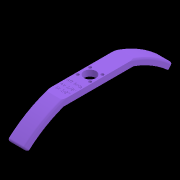
# Autodesk Inventor part: aft_holes
Saved by Autodesk Inventor 2020.2 (Build 242310000, 310)
## iProperties
Created: 2020-04-29
Part Number: aft_holes
Material: PC/ABS Plastic
Document SubType Name: Modeling
Designer: agmlego
Mass: 6.34136 g
Surface Area: 84.683 cm^2
Volume: 17.7494 cm^3
Density: 0.357273 g/cm^3
Appearance: Violet
Author: agmlego
Autodesk Inventor part; units mm, degrees
ref_plane "YZ Plane" through (0, 0, 0) normal (1, 0, 0) x (0, 1, 0)
ref_plane "XZ Plane" through (0, 0, 0) normal (0, 1, 0) x (-1, 0, 0)
ref_plane "XY Plane" through (0, 0, 0) normal (0, 0, 1) x (1, 0, 0)
sketch "Sketch1" plane through (0, 0, 0) normal (1, 0, 0) x (0, 1, 0)
  line L0 (103.1875, 36.7533) -> (103.1875, -36.7533)
  line L1 (109.5375, 37.8345) -> (109.5375, -37.8345)
  line L2 (80.5197, -74.2633) -> (85.1875, -78.5685)
  line L3 (80.5197, 74.2633) -> (85.1875, 78.5685)
  line L4 (85.1875, 78.5685) -> (85.1875, -78.5685) construction
  arc A0 (109.5375, 37.8345) -> (85.1875, 78.5685) centre (0, 0) ccw
  arc A1 (85.1875, -78.5685) -> (109.5375, -37.8345) centre (0, 0) ccw
  arc A2 (103.1875, 36.7533) -> (80.5197, 74.2633) centre (0, 0) ccw
  arc A3 (80.5197, -74.2633) -> (103.1875, -36.7533) centre (0, 0) ccw
  line L5 (109.5375, 0) -> (103.1875, 0) construction
  arc A4 (103.1875, -36.7533) -> (103.1875, 36.7533) centre (0, 0) ccw construction
  dimension "d2" = 6.35
  dimension "d4" = 18
  dimension "d5" = 109.5375
  constraints: 14 end point, 10 point on circle, 5 centre point, 2 coincident, 2 equal length, 2 midpoint, 2 point on line, 1 concentric, 1 horizontal alignment, 1 parallel, 1 perpendicular, 1 tangent, 1 vertical
  measures "d2" distance between parallel lines of L0 L1
  measures "d4" distance between parallel lines of L0 L4
  measures "d5" radius of A2
extrude "Extrusion1" add sketch "Sketch1" along normal blind 18
sketch "Sketch2" plane through (0, 109.5375, 37.8345) normal (0, 1, 0) x (1, 0, 0)
  line L0 (0, 1.0812) -> (0, 74.5878) projected
  line L1 (0, 74.5878) -> (18, 74.5878) projected
  line L2 (18, 1.0812) -> (18, 74.5878) projected
  line L3 (0, 1.0812) -> (18, 1.0812) projected
  line L4 (0, 37.8345) -> (18, 37.8345)
  line L5 (2.5, 44.3345) -> (15.5, 44.3345)
  line L6 (15.5, 44.3345) -> (15.5, 31.3345)
  line L7 (15.5, 31.3345) -> (2.5, 31.3345)
  line L8 (2.5, 31.3345) -> (2.5, 44.3345)
  point P0 (9, 37.8345)
  point P1 (2.5, 37.8345)
  point P2 (9, 44.3345)
  dimension "d8" = 13
  constraints: 10 end point, 4 coincident, 4 midpoint, 2 parallel, 2 perpendicular, 1 horizontal, 1 point on line, 1 vertical alignment
  measures "d8" distance of L5.start L5.end
hole "Hole1" at (2.5, 109.5375, -6.5) at (15.5, 109.5375, -6.5) at (15.5, 109.5375, 6.5) at (2.5, 109.5375, 6.5) direction (0, -1, 0) diameter 3.175 end through all
hole "Hole2" at (9, 109.5375, 0) direction (0, -1, 0) diameter 12.7 end through all
sketch "Sketch3" plane through (0, 109.5375, 37.8345) normal (0, 1, 0) x (1, 0, 0)
  line L0 (0.3251, 23.3588) -> (17.7899, 23.3588) construction
  line L1 (17.7899, 23.3588) -> (17.7899, 6.7355) construction
  line L2 (17.7899, 6.7355) -> (0.3251, 6.7355) construction
  line L3 (0.3251, 6.7355) -> (0.3251, 23.3588) construction
  line L4 (1.3534, 20.1065) -> (2.2041, 22.7156)
  line L5 (2.2041, 22.7156) -> (2.2741, 23.1176)
  line L6 (2.2741, 23.1176) -> (2.7098, 23.1565)
  line L7 (2.7098, 23.1565) -> (3.7083, 20.1065)
  line L8 (3.7083, 20.1065) -> (3.3063, 20.1065)
  line L9 (3.3063, 20.1065) -> (3.0081, 21.009)
  line L10 (3.0081, 21.009) -> (2.0147, 21.009)
  line L11 (2.0147, 21.009) -> (1.7217, 20.1065)
  line L12 (1.7217, 20.1065) -> (1.3534, 20.1065)
  line L13 (2.5127, 22.8349) -> (2.4401, 22.3136)
  line L14 (2.4401, 22.3136) -> (2.1133, 21.3099)
  line L15 (2.1133, 21.3099) -> (2.9121, 21.3099)
  line L16 (2.9121, 21.3099) -> (2.5827, 22.3136)
  line L17 (2.5827, 22.3136) -> (2.5127, 22.8349)
  line L18 (3.9392, 22.3136) -> (4.24, 22.3136)
  line L19 (4.24, 22.3136) -> (4.24, 22.6248)
  spline S0 degree 2 poles (4.24, 22.6248) (4.24, 22.796) (4.3152, 23.0631) (4.4734, 23.2498) (4.725, 23.351) (4.9014, 23.351) knots 0 0 0 1 2 3 4 4 4
  spline S1 degree 2 poles (4.9014, 23.351) (4.9921, 23.351) (5.1426, 23.3199) (5.2696, 23.2732) (5.376, 23.2083) (5.4175, 23.1746) knots 0 0 0 1 2 3 4 4 4
  line L20 (5.4175, 23.1746) -> (5.2463, 22.936)
  spline S2 degree 2 poles (5.2463, 22.936) (5.2048, 22.9671) (5.057, 23.0294) (4.9662, 23.0294) knots 0 0 0 1 2 2 2
  spline S3 degree 2 poles (4.9662, 23.0294) (4.7924, 23.0294) (4.6109, 22.8349) (4.6109, 22.604) knots 0 0 0 1 2 2 2
  line L21 (4.6109, 22.604) -> (4.6109, 22.3136)
  line L22 (4.6109, 22.3136) -> (5.1944, 22.3136)
  line L23 (5.1944, 22.3136) -> (5.1529, 21.992)
  line L24 (5.1529, 21.992) -> (4.6213, 21.992)
  line L25 (4.6213, 21.992) -> (4.6213, 20.1065)
  line L26 (4.6213, 20.1065) -> (4.24, 20.1065)
  line L27 (4.24, 20.1065) -> (4.24, 21.992)
  line L28 (4.24, 21.992) -> (3.9392, 21.992)
  line L29 (3.9392, 21.992) -> (3.9392, 22.3136)
  spline S4 degree 2 poles (6.2267, 20.8612) (6.2267, 20.7289) (6.2578, 20.55) (6.3148, 20.441) (6.4004, 20.3944) (6.4575, 20.3944) knots 0 0 0 1 2 3 4 4 4
  spline S5 degree 2 poles (6.4575, 20.3944) (6.5016, 20.3944) (6.5742, 20.4047) (6.6001, 20.4125) knots 0 0 0 1 2 2 2
  spline S6 degree 2 poles (6.6001, 20.4125) (6.6312, 20.4203) (6.6546, 20.4307) knots 0 0 0 1 1 1
  line L30 (6.6546, 20.4307) -> (6.792, 20.1869)
  spline S7 degree 2 poles (6.792, 20.1869) (6.7765, 20.1713) (6.7065, 20.1324) (6.6105, 20.0961) (6.4886, 20.0728) (6.4186, 20.0728) knots 0 0 0 1 2 3 4 4 4
  spline S8 degree 2 poles (6.4186, 20.0728) (6.237, 20.0728) (6.0114, 20.205) (5.8869, 20.4333) (5.8454, 20.7367) (5.8454, 20.9079) knots 0 0 0 1 2 3 4 4 4
  line L31 (5.8454, 20.9079) -> (5.8454, 21.992)
  line L32 (5.8454, 21.992) -> (5.5446, 21.992)
  line L33 (5.5446, 21.992) -> (5.5446, 22.3136)
  line L34 (5.5446, 22.3136) -> (5.8454, 22.3136)
  line L35 (5.8454, 22.3136) -> (5.8454, 22.7337)
  line L36 (5.8454, 22.7337) -> (6.2163, 22.9568)
  line L37 (6.2163, 22.9568) -> (6.2163, 22.3136)
  line L38 (6.2163, 22.3136) -> (6.8984, 22.3136)
  line L39 (6.8984, 22.3136) -> (6.8595, 21.992)
  line L40 (6.8595, 21.992) -> (6.2267, 21.992)
  line L41 (6.2267, 21.992) -> (6.2267, 20.8612)
  line L42 (9.2378, 20.1065) -> (8.8565, 20.1065)
  line L43 (8.8565, 20.1065) -> (8.8565, 22.9179)
  line L44 (8.8565, 22.9179) -> (8.8176, 23.3199)
  line L45 (8.8176, 23.3199) -> (9.2378, 23.3588)
  line L46 (9.2378, 23.3588) -> (9.2378, 22.0127)
  line L47 (9.2378, 22.0127) -> (9.4167, 22.2461)
  spline S9 degree 2 poles (9.4167, 22.2461) (9.4945, 22.2902) (9.7124, 22.3499) (9.8395, 22.3499) knots 0 0 0 1 2 2 2
  spline S10 degree 2 poles (9.8395, 22.3499) (10.1403, 22.3499) (10.4619, 21.9479) (10.4619, 21.5718) knots 0 0 0 1 2 2 2
  line L48 (10.4619, 21.5718) -> (10.4619, 20.1065)
  line L49 (10.4619, 20.1065) -> (10.0806, 20.1065)
  line L50 (10.0806, 20.1065) -> (10.0806, 21.5303)
  spline S11 degree 2 poles (10.0806, 21.5303) (10.0806, 21.6652) (10.034, 21.8545) (9.951, 21.9738) (9.8265, 22.0283) (9.7487, 22.0283) knots 0 0 0 1 2 3 4 4 4
  spline S12 degree 2 poles (9.7487, 22.0283) (9.6683, 22.0283) (9.5204, 21.9894) (9.3882, 21.9245) (9.2767, 21.8338) (9.2378, 21.7793) knots 0 0 0 1 2 3 4 4 4
  line L51 (9.2378, 21.7793) -> (9.2378, 20.1065)
  spline S13 degree 2 poles (12.0647, 20.0728) (11.8417, 20.0728) (11.476, 20.2465) (11.2114, 20.5552) (11.0636, 20.9753) (11.0636, 21.2165) knots 0 0 0 1 2 3 4 4 4
  spline S14 degree 2 poles (11.0636, 21.2165) (11.0636, 21.4603) (11.2037, 21.8753) (11.4656, 22.1787) (11.8365, 22.3499) (12.0647, 22.3499) knots 0 0 0 1 2 3 4 4 4
  spline S15 degree 2 poles (12.0647, 22.3499) (12.2878, 22.3499) (12.6586, 22.1787) (12.9232, 21.8753) (13.071, 21.4603) (13.071, 21.2165) knots 0 0 0 1 2 3 4 4 4
  spline S16 degree 2 poles (13.071, 21.2165) (13.071, 20.9753) (12.9284, 20.5552) (12.6664, 20.2465) (12.2929, 20.0728) (12.0647, 20.0728) knots 0 0 0 1 2 3 4 4 4
  spline S17 degree 2 poles (12.6897, 21.162) (12.6897, 21.3254) (12.6197, 21.6393) (12.4667, 21.8856) (12.2255, 22.0387) (12.0569, 22.0387) knots 0 0 0 1 2 3 4 4 4
  spline S18 degree 2 poles (12.0569, 22.0387) (11.8961, 22.0387) (11.6627, 21.9064) (11.5149, 21.6859) (11.4449, 21.4032) (11.4449, 21.2554) knots 0 0 0 1 2 3 4 4 4
  spline S19 degree 2 poles (11.4449, 21.2554) (11.4449, 21.092) (11.5149, 20.7808) (11.6653, 20.5344) (11.9039, 20.384) (12.0725, 20.384) knots 0 0 0 1 2 3 4 4 4
  spline S20 degree 2 poles (12.0725, 20.384) (12.2307, 20.384) (12.4641, 20.5163) (12.6171, 20.7367) (12.6897, 21.0168) (12.6897, 21.162) knots 0 0 0 1 2 3 4 4 4
  spline S21 degree 2 poles (14.0565, 20.8612) (14.0565, 20.7289) (14.0877, 20.55) (14.1447, 20.441) (14.2303, 20.3944) (14.2874, 20.3944) knots 0 0 0 1 2 3 4 4 4
  spline S22 degree 2 poles (14.2874, 20.3944) (14.3315, 20.3944) (14.4041, 20.4047) (14.43, 20.4125) knots 0 0 0 1 2 2 2
  spline S23 degree 2 poles (14.43, 20.4125) (14.4611, 20.4203) (14.4845, 20.4307) knots 0 0 0 1 1 1
  line L52 (14.4845, 20.4307) -> (14.6219, 20.1869)
  spline S24 degree 2 poles (14.6219, 20.1869) (14.6064, 20.1713) (14.5363, 20.1324) (14.4404, 20.0961) (14.3185, 20.0728) (14.2485, 20.0728) knots 0 0 0 1 2 3 4 4 4
  spline S25 degree 2 poles (14.2485, 20.0728) (14.0669, 20.0728) (13.8413, 20.205) (13.7168, 20.4333) (13.6753, 20.7367) (13.6753, 20.9105) knots 0 0 0 1 2 3 4 4 4
  line L53 (13.6753, 20.9105) -> (13.6753, 22.9179)
  line L54 (13.6753, 22.9179) -> (13.6364, 23.3199)
  line L55 (13.6364, 23.3199) -> (14.0565, 23.3588)
  line L56 (14.0565, 23.3588) -> (14.0565, 20.8612)
  spline S26 degree 2 poles (16.6164, 20.3658) (16.5541, 20.301) (16.4063, 20.1947) (16.2247, 20.1143) (16.0069, 20.0728) (15.872, 20.0728) knots 0 0 0 1 2 3 4 4 4
  spline S27 degree 2 poles (15.872, 20.0728) (15.6049, 20.0728) (15.2288, 20.2621) (14.9902, 20.5785) (14.8787, 20.9883) (14.8787, 21.2113) knots 0 0 0 1 2 3 4 4 4
  spline S28 degree 2 poles (14.8787, 21.2113) (14.8787, 21.354) (14.9306, 21.6341) (15.0343, 21.8856) (15.1925, 22.1035) (15.4, 22.2591) (15.6645, 22.3499) (15.8227, 22.3499) knots 0 0 0 1 2 3 4 5 6 6 6
  spline S29 degree 2 poles (15.8227, 22.3499) (16.038, 22.3499) (16.357, 22.2098) (16.5645, 21.9557) (16.6656, 21.6029) (16.6656, 21.3877) knots 0 0 0 1 2 3 4 4 4
  spline S30 degree 2 poles (16.6656, 21.3877) (16.6656, 21.3254) (16.6579, 21.1776) (16.6501, 21.1102) knots 0 0 0 1 2 2 2
  line L57 (16.6501, 21.1102) -> (15.2599, 21.1102)
  spline S31 degree 2 poles (15.2599, 21.1102) (15.2599, 20.9597) (15.3429, 20.7004) (15.4908, 20.5059) (15.7008, 20.3944) (15.8331, 20.3944) knots 0 0 0 1 2 3 4 4 4
  spline S32 degree 2 poles (15.8331, 20.3944) (15.9602, 20.3944) (16.1521, 20.4333) (16.287, 20.4877) (16.3752, 20.5422) (16.3985, 20.5577) knots 0 0 0 1 2 3 4 4 4
  line L58 (16.3985, 20.5577) -> (16.6164, 20.3658)
  spline S33 degree 2 poles (16.2844, 21.411) (16.287, 21.4344) (16.2896, 21.4785) (16.2896, 21.4992) knots 0 0 0 1 2 2 2
  spline S34 degree 2 poles (16.2896, 21.4992) (16.2896, 21.6133) (16.2351, 21.8078) (16.1288, 21.9505) (15.9654, 22.0309) (15.8513, 22.0309) knots 0 0 0 1 2 3 4 4 4
  spline S35 degree 2 poles (15.8513, 22.0309) (15.719, 22.0309) (15.5271, 21.9453) (15.3974, 21.8104) (15.317, 21.6496) (15.2988, 21.577) knots 0 0 0 1 2 3 4 4 4
  line L59 (15.2988, 21.577) -> (15.1925, 21.3566)
  line L60 (15.1925, 21.3566) -> (15.5504, 21.411)
  line L61 (15.5504, 21.411) -> (16.2844, 21.411)
  line L62 (3.6098, 13.985) -> (3.2493, 13.985)
  line L63 (3.2493, 13.985) -> (3.2493, 13.3833)
  line L64 (3.2493, 13.3833) -> (2.8265, 13.3833)
  line L65 (2.8265, 13.3833) -> (2.8265, 13.985)
  line L66 (2.8265, 13.985) -> (1.6309, 13.985)
  line L67 (1.6309, 13.985) -> (1.6309, 14.3274)
  line L68 (1.6309, 14.3274) -> (2.6035, 16.4333)
  line L69 (2.6035, 16.4333) -> (2.9847, 16.3944)
  line L70 (2.9847, 16.3944) -> (2.1496, 14.5867)
  line L71 (2.1496, 14.5867) -> (1.9629, 14.3066)
  line L72 (1.9629, 14.3066) -> (2.8265, 14.3066)
  line L73 (2.8265, 14.3066) -> (2.8265, 15.1236)
  line L74 (2.8265, 15.1236) -> (3.2493, 15.0899)
  line L75 (3.2493, 15.0899) -> (3.2493, 14.3066)
  line L76 (3.2493, 14.3066) -> (3.6409, 14.3066)
  line L77 (3.6409, 14.3066) -> (3.6098, 13.985)
  line L78 (5.7494, 13.3833) -> (5.21, 14.151)
  line L79 (5.21, 14.151) -> (5.1218, 14.387)
  line L80 (5.1218, 14.387) -> (5.031, 14.151)
  line L81 (5.031, 14.151) -> (4.4916, 13.3833)
  line L82 (4.4916, 13.3833) -> (4.0922, 13.3833)
  line L83 (4.0922, 13.3833) -> (4.9195, 14.5634)
  line L84 (4.9195, 14.5634) -> (4.2011, 15.593)
  line L85 (4.2011, 15.593) -> (4.6238, 15.6267)
  line L86 (4.6238, 15.6267) -> (5.0959, 14.9524)
  line L87 (5.0959, 14.9524) -> (5.1763, 14.7294)
  line L88 (5.1763, 14.7294) -> (5.2515, 14.9524)
  line L89 (5.2515, 14.9524) -> (5.7028, 15.593)
  line L90 (5.7028, 15.593) -> (6.1255, 15.6267)
  line L91 (6.1255, 15.6267) -> (5.376, 14.553)
  line L92 (5.376, 14.553) -> (6.2007, 13.3833)
  line L93 (6.2007, 13.3833) -> (5.7494, 13.3833)
  line L94 (8.3534, 13.3833) -> (8.3534, 13.7049)
  line L95 (8.3534, 13.7049) -> (8.8461, 13.7049)
  line L96 (8.8461, 13.7049) -> (8.8461, 15.6423)
  line L97 (8.8461, 15.6423) -> (8.9628, 16.0988)
  line L98 (8.9628, 16.0988) -> (8.6905, 15.7253)
  line L99 (8.6905, 15.7253) -> (8.2652, 15.3492)
  line L100 (8.2652, 15.3492) -> (8.0473, 15.5904)
  line L101 (8.0473, 15.5904) -> (8.968, 16.4333)
  line L102 (8.968, 16.4333) -> (9.2689, 16.3944)
  line L103 (9.2689, 16.3944) -> (9.2689, 13.7049)
  line L104 (9.2689, 13.7049) -> (9.7616, 13.7049)
  line L105 (9.7616, 13.7049) -> (9.7616, 13.3833)
  line L106 (9.7616, 13.3833) -> (8.3534, 13.3833)
  line L107 (10.8354, 13.1836) -> (10.4126, 13.1836)
  line L108 (10.4126, 13.1836) -> (11.8391, 16.5941)
  line L109 (11.8391, 16.5941) -> (12.2385, 16.5941)
  line L110 (12.2385, 16.5941) -> (10.8354, 13.1836)
  spline S36 degree 2 poles (13.696, 16.4281) (13.8802, 16.4281) (14.194, 16.327) (14.4196, 16.1402) (14.5493, 15.8705) (14.5493, 15.7019) knots 0 0 0 1 2 3 4 4 4
  spline S37 degree 2 poles (14.5493, 15.7019) (14.5493, 15.5826) (14.4793, 15.3985) (14.3574, 15.2533) (14.1992, 15.134) (14.111, 15.0821) knots 0 0 0 1 2 3 4 4 4
  spline S38 degree 2 poles (14.111, 15.0821) (14.2588, 15.0147) (14.4949, 14.8435) (14.6582, 14.6308) (14.7438, 14.3663) (14.7438, 14.2055) knots 0 0 0 1 2 3 4 4 4
  spline S39 degree 2 poles (14.7438, 14.2055) (14.7438, 13.985) (14.5675, 13.6608) (14.277, 13.4507) (13.9035, 13.3496) (13.709, 13.3496) knots 0 0 0 1 2 3 4 4 4
  spline S40 degree 2 poles (13.709, 13.3496) (13.5171, 13.3496) (13.1644, 13.4637) (12.8946, 13.6868) (12.7287, 14.0187) (12.7287, 14.234) knots 0 0 0 1 2 3 4 4 4
  spline S41 degree 2 poles (12.7287, 14.234) (12.7287, 14.3948) (12.822, 14.6567) (12.9828, 14.8642) (13.2033, 15.0276) (13.3304, 15.0899) knots 0 0 0 1 2 3 4 4 4
  spline S42 degree 2 poles (13.3304, 15.0899) (13.237, 15.1469) (13.0736, 15.2714) (12.9517, 15.4141) (12.8817, 15.58) (12.8817, 15.6786) knots 0 0 0 1 2 3 4 4 4
  spline S43 degree 2 poles (12.8817, 15.6786) (12.8817, 15.8731) (13.0373, 16.1584) (13.2785, 16.3399) (13.5638, 16.4281) (13.696, 16.4281) knots 0 0 0 1 2 3 4 4 4
  spline S44 degree 2 poles (13.6727, 14.9083) (13.5456, 14.8564) (13.3433, 14.7242) (13.2007, 14.5582) (13.1229, 14.3507) (13.1229, 14.2158) knots 0 0 0 1 2 3 4 4 4
  spline S45 degree 2 poles (13.1229, 14.2158) (13.1229, 14.0939) (13.2214, 13.8968) (13.3848, 13.7542) (13.5975, 13.679) (13.709, 13.679) knots 0 0 0 1 2 3 4 4 4
  spline S46 degree 2 poles (13.709, 13.679) (13.8387, 13.679) (14.0695, 13.749) (14.2433, 13.8865) (14.3444, 14.0862) (14.3444, 14.2158) knots 0 0 0 1 2 3 4 4 4
  spline S47 degree 2 poles (14.3444, 14.2158) (14.3444, 14.3507) (14.2251, 14.5634) (14.0358, 14.7294) (13.7972, 14.8564) (13.6727, 14.9083) knots 0 0 0 1 2 3 4 4 4
  spline S48 degree 2 poles (13.7583, 15.2351) (13.9424, 15.3181) (14.1629, 15.5515) (14.1629, 15.7175) knots 0 0 0 1 2 2 2
  spline S49 degree 2 poles (14.1629, 15.7175) (14.1629, 15.8186) (14.0799, 15.9613) (13.9554, 16.0547) (13.8024, 16.0962) (13.7349, 16.0962) knots 0 0 0 1 2 3 4 4 4
  spline S50 degree 2 poles (13.7349, 16.0962) (13.6442, 16.0962) (13.4756, 16.0417) (13.3459, 15.9405) (13.2681, 15.8057) (13.2681, 15.7253) knots 0 0 0 1 2 3 4 4 4
  spline S51 degree 2 poles (13.2681, 15.7253) (13.2681, 15.6319) (13.3459, 15.4919) (13.4808, 15.3777) (13.6597, 15.2792) (13.7583, 15.2351) knots 0 0 0 1 2 3 4 4 4
  line L111 (16.3337, 16.3944) -> (16.3337, 16.1947)
  spline S52 degree 2 poles (16.3337, 16.1947) (16.3337, 16.1169) (16.3051, 15.8939) (16.2896, 15.7849) knots 0 0 0 1 2 2 2
  spline S53 degree 2 poles (16.2896, 15.7849) (16.2688, 15.6604) (16.2455, 15.5256) knots 0 0 0 1 1 1
  line L112 (16.2455, 15.5256) -> (16.0717, 15.5256)
  spline S54 degree 2 poles (16.0717, 15.5256) (16.0484, 15.6604) (16.0276, 15.7849) knots 0 0 0 1 1 1
  spline S55 degree 2 poles (16.0276, 15.7849) (16.0121, 15.8939) (15.9835, 16.1169) (15.9835, 16.1947) knots 0 0 0 1 2 2 2
  line L113 (15.9835, 16.1947) -> (15.9835, 16.3944)
  line L114 (15.9835, 16.3944) -> (16.3337, 16.3944)
  line L115 (15.7294, 16.3944) -> (15.7294, 16.1947)
  spline S56 degree 2 poles (15.7294, 16.1947) (15.7294, 16.1169) (15.7008, 15.8939) (15.6853, 15.7849) knots 0 0 0 1 2 2 2
  spline S57 degree 2 poles (15.6853, 15.7849) (15.6645, 15.6604) (15.6412, 15.5256) knots 0 0 0 1 1 1
  line L116 (15.6412, 15.5256) -> (15.4674, 15.5256)
  spline S58 degree 2 poles (15.4674, 15.5256) (15.4441, 15.6604) (15.4233, 15.7849) knots 0 0 0 1 1 1
  spline S59 degree 2 poles (15.4233, 15.7849) (15.4078, 15.8939) (15.3792, 16.1169) (15.3792, 16.1947) knots 0 0 0 1 2 2 2
  line L117 (15.3792, 16.1947) -> (15.3792, 16.3944)
  line L118 (15.3792, 16.3944) -> (15.7294, 16.3944)
  line L119 (4.241, 7.3975) -> (2.754, 7.3975)
  line L120 (2.754, 7.3975) -> (2.754, 7.7087)
  line L121 (2.754, 7.7087) -> (3.3073, 7.7087)
  line L122 (3.3073, 7.7087) -> (3.3073, 9.7514)
  line L123 (3.3073, 9.7514) -> (2.754, 9.7514)
  line L124 (2.754, 9.7514) -> (2.754, 10.0305)
  spline S60 degree 2 poles (2.754, 10.0305) (3.0677, 10.0305) (3.3641, 10.2084) (3.3839, 10.4554) knots 0 0 0 1 2 2 2
  line L125 (3.3839, 10.4554) -> (3.7, 10.4554)
  line L126 (3.7, 10.4554) -> (3.7, 7.7087)
  line L127 (3.7, 7.7087) -> (4.241, 7.7087)
  line L128 (4.241, 7.7087) -> (4.241, 7.3975)
  line L129 (6.6344, 7.3975) -> (6.1626, 7.3975)
  line L130 (6.1626, 7.3975) -> (5.6069, 8.2571)
  line L131 (5.6069, 8.2571) -> (5.0363, 7.3975)
  line L132 (5.0363, 7.3975) -> (4.5991, 7.3975)
  line L133 (4.5991, 7.3975) -> (5.392, 8.5312)
  line L134 (5.392, 8.5312) -> (4.6065, 9.6847)
  line L135 (4.6065, 9.6847) -> (5.0783, 9.6847)
  line L136 (5.0783, 9.6847) -> (5.6316, 8.8326)
  line L137 (5.6316, 8.8326) -> (6.1972, 9.6847)
  line L138 (6.1972, 9.6847) -> (6.6344, 9.6847)
  line L139 (6.6344, 9.6847) -> (5.8465, 8.5559)
  line L140 (5.8465, 8.5559) -> (6.6344, 7.3975)
  line L141 (9.9121, 7.3975) -> (8.4252, 7.3975)
  line L142 (8.4252, 7.3975) -> (8.4252, 7.7087)
  line L143 (8.4252, 7.7087) -> (8.9785, 7.7087)
  line L144 (8.9785, 7.7087) -> (8.9785, 9.7514)
  line L145 (8.9785, 9.7514) -> (8.4252, 9.7514)
  line L146 (8.4252, 9.7514) -> (8.4252, 10.0305)
  spline S61 degree 2 poles (8.4252, 10.0305) (8.7389, 10.0305) (9.0353, 10.2084) (9.055, 10.4554) knots 0 0 0 1 2 2 2
  line L147 (9.055, 10.4554) -> (9.3712, 10.4554)
  line L148 (9.3712, 10.4554) -> (9.3712, 7.7087)
  line L149 (9.3712, 7.7087) -> (9.9121, 7.7087)
  line L150 (9.9121, 7.7087) -> (9.9121, 7.3975)
  line L151 (11.7399, 10.5814) -> (10.5469, 6.7355)
  line L152 (10.5469, 6.7355) -> (10.2011, 6.7355)
  line L153 (10.2011, 6.7355) -> (11.3892, 10.5814)
  line L154 (11.3892, 10.5814) -> (11.7399, 10.5814)
  line L155 (13.9555, 7.3975) -> (12.0759, 7.3975)
  line L156 (12.0759, 7.3975) -> (12.0759, 7.8298)
  spline S62 degree 2 poles (12.0759, 7.8298) (12.2784, 8.0199) (12.639, 8.3732) (12.8119, 8.5634) knots 0 0 0 1 2 2 2
  spline S63 degree 2 poles (12.8119, 8.5634) (13.1602, 8.9462) (13.4146, 9.4056) (13.4146, 9.6502) knots 0 0 0 1 2 2 2
  spline S64 degree 2 poles (13.4146, 9.6502) (13.4146, 9.7786) (13.3356, 9.9713) (13.2639, 10.033) knots 0 0 0 1 2 2 2
  spline S65 degree 2 poles (13.2639, 10.033) (13.1923, 10.0948) (13.0046, 10.1565) (12.891, 10.1565) knots 0 0 0 1 2 2 2
  spline S66 degree 2 poles (12.891, 10.1565) (12.7823, 10.1565) (12.56, 10.1022) (12.4587, 10.0602) knots 0 0 0 1 2 2 2
  spline S67 degree 2 poles (12.4587, 10.0602) (12.3723, 10.0256) (12.2117, 9.9268) (12.1623, 9.8922) knots 0 0 0 1 2 2 2
  line L157 (12.1623, 9.8922) -> (12.1401, 9.8922)
  line L158 (12.1401, 9.8922) -> (12.1401, 10.3269)
  spline S68 degree 2 poles (12.1401, 10.3269) (12.2661, 10.3887) (12.7181, 10.5097) (12.9206, 10.5097) knots 0 0 0 1 2 2 2
  spline S69 degree 2 poles (12.9206, 10.5097) (13.3479, 10.5097) (13.8296, 10.0577) (13.8296, 9.6724) knots 0 0 0 1 2 2 2
  spline S70 degree 2 poles (13.8296, 9.6724) (13.8296, 9.4921) (13.7456, 9.1907) (13.6715, 9.0623) knots 0 0 0 1 2 2 2
  spline S71 degree 2 poles (13.6715, 9.0623) (13.5974, 8.9289) (13.3825, 8.6671) (13.2639, 8.5411) knots 0 0 0 1 2 2 2
  spline S72 degree 2 poles (13.2639, 8.5411) (13.0713, 8.3312) (12.5995, 7.8816) (12.4587, 7.7507) knots 0 0 0 1 2 2 2
  line L159 (12.4587, 7.7507) -> (13.9555, 7.7507)
  line L160 (13.9555, 7.7507) -> (13.9555, 7.3975)
  line L161 (14.82, 10.5814) -> (14.7311, 9.3957)
  line L162 (14.7311, 9.3957) -> (14.4619, 9.3957)
  line L163 (14.4619, 9.3957) -> (14.373, 10.5814)
  line L164 (14.373, 10.5814) -> (14.82, 10.5814)
  line L165 (15.5907, 10.5814) -> (15.5018, 9.3957)
  line L166 (15.5018, 9.3957) -> (15.2325, 9.3957)
  line L167 (15.2325, 9.3957) -> (15.1436, 10.5814)
  line L168 (15.1436, 10.5814) -> (15.5907, 10.5814)
  point P0 (0, 37.8345)
  constraints: 2 other
emboss "Emboss1" sketch "Sketch3" operation cut depth 1 direction (0, -1, 0)
fillet "Fillet1" radius 2 12 edges at (9, 85.1875, 78.5685) (9, 80.5197, 74.2633) (18, 82.8536, 76.4159) (0, 82.8536, 76.4159) (9, 85.1875, -78.5685) (0, 82.8536, -76.4159) (9, 80.5197, -74.2633) (18, 82.8536, -76.4159) (18, 99.4699, 59.4613) (0, 99.4699, 59.4613) (18, 99.4699, -59.4613) (0, 99.4699, -59.4613)
equation "\"d5\" = 0.5 * hull_od"
equation "\"hull_od\" = 219.075"
equation "\"hull_id\" = 201.7268"
equation "\"hull_wall\" = 8.6741"
equation "\"hull_length\" = 609.6"
equation "\"hull_spacing\" = 390.525"
equation "\"impeller_od\" = 76.2"
equation "\"impeller_clearance\" = 0.5"
equation "\"impeller_shaft_id\" = 3.175"
equation "\"impeller_shaft_od\" = 5.715"
equation "\"impeller_shaft_support\" = 3.175"
equation "\"impeller_intake_od\" = 19.05"
equation "\"impeller_vane_thick\" = 2"
equation "\"impeller_vane_inner_rad\" = 3.175"
equation "\"impeller_vane_outer_rad\" = 0.37206"
equation "\"magnet_od\" = 5.95"
equation "\"magnet_clearance\" = 0.25"
equation "\"magnet_rad\" = 0.25"
equation "\"magnet_circle_offset\" = 3.175"
equation "\"motor_shaft_od\" = 12.7"
equation "\"motor_shaft_length\" = 31.75"
equation "\"motor_shaft_key\" = 3.048"
equation "\"slab_thick\" = 34.671"
equation "\"d0\" = hull_od"
equation "\"d3\" = d2"
body "Solid1"
